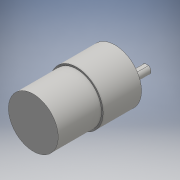
# Autodesk Inventor part: 37D mm metal gearmotor
Saved by Autodesk Inventor 2016 (Build 200138000, 138)
## iProperties
Created: 2016-05-11
Part Number: 37D mm metal gearmotor
Material: Generic
Document SubType Name: Modeling
Designer: hesaon
Density: 1 g/cm^3
Appearance: Default
Author: hesaon
Autodesk Inventor part; units mm, degrees
ref_plane "YZ Plane" through (0, 0, 0) normal (1, 0, 0) x (0, 1, 0)
ref_plane "XZ Plane" through (0, 0, 0) normal (0, 1, 0) x (-1, 0, 0)
ref_plane "XY Plane" through (0, 0, 0) normal (0, 0, 1) x (1, 0, 0)
sketch "Sketch1" plane through (0, 0, 0) normal (0, 1, 0) x (-1, 0, 0)
  circle A0 centre (0, 0) radius 18.4
  dimension "d0" = 36.8
  constraints: 1 centre point, 1 coincident
  measures "d0" diameter of A0
sketch "Sketch1 outline for Extrusion1" plane through (0, 0, 0) normal (0, 1, 0) x (-1, 0, 0)
  circle A0 centre (0, 0) radius 18.4
extrude "Extrusion1" add sketch "Sketch1 outline for Extrusion1" along normal blind 26.6
sketch "Sketch2" plane through (0, 26.6, 0) normal (0, 1, 0) x (1, 0, 0)
  circle A0 centre (0, 7) radius 6
  point P0 (0, 0)
  dimension "d5" = 0
  dimension "d6" = 7
  dimension "d7" = 12
  constraints: 1 centre point, 1 coincident
  measures "d5" horizontal distance of point (0, 0) point (0, 7)
  measures "d6" distance of point (0, 0) point (0, 7)
  measures "d7" diameter of A0
sketch "Sketch2 outline for Extrusion2" plane through (0, 26.6, 0) normal (0, 1, 0) x (1, 0, 0)
  circle A0 centre (0, 7) radius 6
extrude "Extrusion2" add sketch "Sketch2 outline for Extrusion2" along normal blind 6.5
chamfer "Chamfer1" distance 0.5 angle 45 1 edges at (-6, 33.1, -7)
sketch "Sketch3" plane through (0, 26.6, 0) normal (0, 1, 0) x (1, 0, 0)
  circle A0 centre (0, 0) radius 18.4
  circle A1 centre (0, 0) radius 18.4
  arc A2 (-8.477201, 7.622143) -> (8.477201, 7.622143) centre (0, 7) ccw
  arc A3 (-8.477201, 7.622143) -> (8.477201, 7.622143) centre (0, 0) ccw
  dimension "d13" = 0
  dimension "d14" = 7
  dimension "d15" = 17
  dimension "d16" = 22.8
  constraints: 4 point on circle, 3 coincident, 2 centre point
  measures "d13" horizontal distance of A0.centre point (0, 7)
  measures "d14" distance of point (0, 0) point (0, 7)
  measures "d15" diameter of A2
  measures "d16" diameter of A3
sketch "Sketch3 outline for Extrusion3" plane through (0, 26.6, 0) normal (0, 1, 0) x (1, 0, 0)
  arc A0 (-8.477201, 7.622143) -> (8.477201, 7.622143) centre (0, 0) ccw
  arc A1 (8.477201, 7.622143) -> (-8.477201, 7.622143) centre (0, 7) cw
extrude "Extrusion3" cut sketch "Sketch3 outline for Extrusion3" against normal blind 1
chamfer "Chamfer3" distance 1 angle 45 2 edges at (0, 26.6, 11.4) (0, 26.6, 1.5)
sketch "Sketch4" plane through (0, 33.1, -7) normal (0, 1, 0) x (1, 0, 0)
  circle A0 centre (0, 0) radius 3
  circle A1 centre (0, 0) radius 6 projected
  point P0 (0, -7)
  dimension "d25" = 6
  constraints: 1 centre point, 1 concentric
  measures "d25" diameter of A0
sketch "Sketch4 outline for Extrusion4" plane through (0, 33.1, -7) normal (0, 1, 0) x (1, 0, 0)
  circle A0 centre (0, 0) radius 3
extrude "Extrusion4" add sketch "Sketch4 outline for Extrusion4" along normal blind 15.5
sketch "Sketch5" plane through (0, 48.6, -7) normal (0, 1, 0) x (1, 0, 0)
  line L0 (0, -2.7) -> (-1.30767, -2.7)
  line L1 (0, -2.7) -> (1.30767, -2.7)
  circle A0 centre (0, 0) radius 3
  arc A1 (-1.30767, -2.7) -> (1.30767, -2.7) centre (0, 0) ccw
  point P0 (0, -7)
  dimension "d33" = 4.3
  constraints: 4 end point, 2 horizontal, 2 point on circle, 1 centre point, 1 coincident
  measures "d33" distance of point (0, -7) L0.start
sketch "Sketch5 outline for Extrusion5" plane through (0, 48.6, -7) normal (0, 1, 0) x (1, 0, 0)
  line L0 (1.30767, -2.7) -> (0, -2.7)
  arc A0 (-1.30767, -2.7) -> (1.30767, -2.7) centre (0, 0) ccw
  line L1 (0, -2.7) -> (-1.30767, -2.7)
extrude "Extrusion5" cut sketch "Sketch5 outline for Extrusion5" against normal blind 12
sketch "Sketch6" plane through (0, 0, 0) normal (0, -1, 0) x (1, 0, 0)
  circle A0 centre (0, 0) radius 17.25
  dimension "d36" = 34.5
  constraints: 1 centre point, 1 coincident
  measures "d36" diameter of A0
sketch "Sketch6 outline for Extrusion6" plane through (0, 0, 0) normal (0, -1, 0) x (1, 0, 0)
  circle A0 centre (0, 0) radius 17.25
extrude "Extrusion6" add sketch "Sketch6 outline for Extrusion6" along normal blind 30
body "Solid1"
